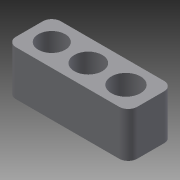
# Autodesk Inventor part: 6mmHoleTest6-6.25-6.5mm
Saved by Autodesk Inventor 2014 SP1 (Build 180222100, 222)
## iProperties
Created: 2016-11-29
Part Number: 6mmHoleTest6-6.25-6.5mm
Material: Generic
Document SubType Name: Modeling
Designer: danielsikar
Density: 1 g/cm^3
Appearance: Default
Author: danielsikar
Autodesk Inventor part; units mm, degrees
ref_plane "YZ Plane" through (0, 0, 0) normal (1, 0, 0) x (0, 1, 0)
ref_plane "XZ Plane" through (0, 0, 0) normal (0, 1, 0) x (-1, 0, 0)
ref_plane "XY Plane" through (0, 0, 0) normal (0, 0, 1) x (1, 0, 0)
sketch "Sketch1" plane through (0, 0, 0) normal (0, 0, 1) x (1, 0, 0)
  line L0 (27, 1) -> (27, 11)
  line L1 (0, 11) -> (0, 1)
  circle A0 centre (5, 6) radius 3
  circle A1 centre (13.125, 6) radius 3.125
  circle A2 centre (21.5, 6) radius 3.25
  line L2 (0, 11) -> (27, 11)
  line L3 (0, 1) -> (27, 1)
  point P0 (0, 0)
  dimension "d2" = 6
  dimension "d3" = 6.25
  dimension "d4" = 6.5
  dimension "d7" = 8.375
  dimension "d8" = 5
  dimension "d9" = 5
  constraints: 8 end point, 3 centre point, 2 parallel, 1 perpendicular
  measures "d2" diameter of A0
  measures "d3" diameter of A1
  measures "d4" diameter of A2
  measures "d7" distance of A1.centre A2.centre
  measures "d8" distance from line of A0.centre L3
  measures "d9" distance from line of L2 A0.centre
extrude "Extrusion1" add sketch "Sketch1" along normal blind 10
fillet "Fillet1" radius 2 4 edges at (0, 11, 5) (27, 11, 5) (27, 1, 5) (0, 1, 5)
body "Solid1"
